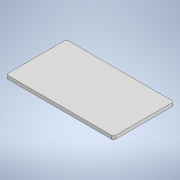
# Autodesk Inventor part: front
Saved by Autodesk Inventor 2021 (Build 250183000, 183)
## iProperties
Created: 2025-12-27
Part Number: front
Material: Generic
Description: FreeCAD Model
Document SubType Name: Modeling
Designer: Ignacio
Authority: Unknown
Density: 1 g/cm^3
Appearance: Default
Sending System: FreeCAD
Preprocessor: Open CASCADE STEP processor 7.6
Title: Open CASCADE Shape Model
Autodesk Inventor part; units mm, degrees
ref_plane "YZ Plane" through (0, 0, 0) normal (1, 0, 0) x (0, 1, 0)
ref_plane "XZ Plane" through (0, 0, 0) normal (0, 1, 0) x (-1, 0, 0)
ref_plane "XY Plane" through (0, 0, 0) normal (0, 0, 1) x (1, 0, 0)
sketch "Sketch2" plane through (0, 0, 0) normal (0, 1, 0) x (-1, 0, 0)
  line L0 (0, 0) -> (125.1, 0)
  line L1 (125.1, 0) -> (125.1, -70.1)
  line L2 (125.1, -70.1) -> (0, -70.1)
  line L3 (0, -70.1) -> (0, 0)
  dimension "d5" = 70.1
  dimension "d6" = 125.1
  constraints: 8 end point, 2 parallel, 1 horizontal, 1 perpendicular
  measures "d5" distance of L0.end L1.end
  measures "d6" distance of L1.end L2.end
extrude "Extrusion2" add sketch "Sketch2" along normal blind 4
fillet "Fillet1" radius 2 4 edges at (-125.1, 2, 0) (-125.1, 2, -70.1) (0, 2, 0) (0, 2, -70.1)
body "Solid2"
